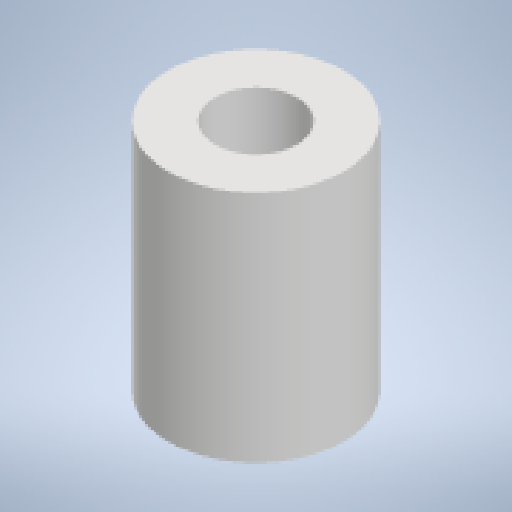
# Autodesk Inventor part: втулка
Saved by Autodesk Inventor 2024.2 (Build 282272000, 272)
## iProperties
Created: 2023-08-07
Part Number: втулка
Material: Generic
Document SubType Name: Modeling
Designer: admin
Density: 1 g/cm^3
Appearance: Default
Author: admin
Autodesk Inventor part; units mm, degrees
ref_plane "YZ Plane" through (0, 0, 0) normal (1, 0, 0) x (0, 1, 0)
ref_plane "XZ Plane" through (0, 0, 0) normal (0, 1, 0) x (-1, 0, 0)
ref_plane "XY Plane" through (0, 0, 0) normal (0, 0, 1) x (1, 0, 0)
sketch "Sketch1" plane through (0, 0, 0) normal (0, 0, 1) x (1, 0, 0)
  line L0 (0, 20) -> (0, -20)
  line L1 (0, -20) -> (7, -20) construction
  line L2 (0, 20) -> (7, 20) construction
  line L3 (15, 20) -> (15, -20)
  line L4 (7, 20) -> (7, -20)
  line L5 (7, 20) -> (15, 20)
  line L6 (7, -20) -> (15, -20)
  point P0 (0, 0)
  point P1 (0, 0)
  dimension "d18" = 40
  dimension "d19" = 30
  dimension "d43" = 14
  constraints: 15 end point, 4 perpendicular, 2 horizontal, 2 midpoint, 2 vertical, 1 coincident
  measures "d18" distance of L3.start L3.end
  measures "d19" diameter of L3 L0
  measures "d43" diameter of L4 L0
revolve "Revolution1" add sketch "Sketch1" angle 360 about axis through (0, 20, 0) along (0, -1, 0)
body "Solid1"
